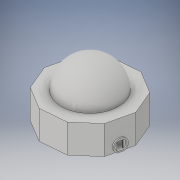
# Autodesk Inventor part: dome
Saved by Autodesk Inventor 2017 (Build 210142000, 142)
## iProperties
Created: 2018-03-05
Part Number: dome
Material: Generic
Document SubType Name: Modeling
Designer: Braxton
Density: 1 g/cm^3
Appearance: Default
Author: Braxton
Autodesk Inventor part; units mm, degrees
ref_plane "YZ Plane" through (0, 0, 0) normal (1, 0, 0) x (0, 1, 0)
ref_plane "XZ Plane" through (0, 0, 0) normal (0, 1, 0) x (-1, 0, 0)
ref_plane "XY Plane" through (0, 0, 0) normal (0, 0, 1) x (1, 0, 0)
sketch "Sketch1" plane through (0, 0, 0) normal (0, 1, 0) x (-1, 0, 0)
  line L0 (707.6587, -429.7359) -> (319.9155, -763.615)
  line L1 (319.9155, -763.615) -> (-190.0245, -805.8191)
  line L2 (-190.0245, -805.8191) -> (-627.3817, -540.2278)
  line L3 (-627.3817, -540.2278) -> (-825.1003, -68.2877)
  line L4 (-825.1003, -68.2877) -> (-707.6587, 429.7359)
  line L5 (-707.6587, 429.7359) -> (-319.9155, 763.615)
  line L6 (-319.9155, 763.615) -> (190.0245, 805.8191)
  line L7 (190.0245, 805.8191) -> (627.3817, 540.2278)
  line L8 (627.3817, 540.2278) -> (825.1003, 68.2877)
  line L9 (825.1003, 68.2877) -> (707.6587, -429.7359)
  point P0 (0, 0)
  point P1 (0, 0)
  dimension "d0" = 1574.8
  constraints: 20 end point, 1 coincident, 21 other
  measures "d0" distance between parallel lines of L5 L0
extrude "bace" add sketch "Sketch1" along normal blind 25.4
sketch "Sketch2" plane through (0, 25.4, 0) normal (0, 1, 0) x (1, 0, 0)
  line L0 (-319.9155, 763.615) -> (-707.6587, 429.7359) projected
  line L1 (-707.6587, 429.7359) -> (-319.9155, 763.615)
  line L2 (-319.9155, 763.615) -> (190.0245, 805.8191)
  line L3 (190.0245, 805.8191) -> (627.3817, 540.2278)
  line L4 (627.3817, 540.2278) -> (825.1003, 68.2877)
  line L5 (825.1003, 68.2877) -> (707.6587, -429.7359)
  line L6 (707.6587, -429.7359) -> (319.9155, -763.615)
  line L7 (319.9155, -763.615) -> (-190.0245, -805.8191)
  line L8 (-190.0245, -805.8191) -> (-627.3817, -540.2278)
  line L9 (-627.3817, -540.2278) -> (-825.1003, -68.2877)
  line L10 (-825.1003, -68.2877) -> (-707.6587, 429.7359)
  line L11 (-684.831, 415.8734) -> (-309.5957, 738.9822)
  line L12 (-309.5957, 738.9822) -> (183.8947, 779.825)
  line L13 (183.8947, 779.825) -> (607.1435, 522.8011)
  line L14 (607.1435, 522.8011) -> (798.4842, 66.0849)
  line L15 (798.4842, 66.0849) -> (684.831, -415.8734)
  line L16 (684.831, -415.8734) -> (309.5957, -738.9822)
  line L17 (309.5957, -738.9822) -> (-183.8947, -779.825)
  line L18 (-183.8947, -779.825) -> (-607.1435, -522.8011)
  line L19 (-607.1435, -522.8011) -> (-798.4842, -66.0849)
  line L20 (-798.4842, -66.0849) -> (-684.831, 415.8734)
  line L21 (-707.6587, 429.7359) -> (-825.1003, -68.2877) projected
  point P0 (0, 0)
  point P1 (0, 0)
  point P2 (0, 0)
  dimension "d4" = 25.4
  constraints: 40 end point, 2 coincident, 1 parallel, 42 other
  measures "d4" distance between parallel lines of L21 L20
extrude "bace wall" add sketch "Sketch2" along normal blind 508
sketch "Sketch3" plane through (0, 533.4, 0) normal (0, 1, 0) x (1, 0, 0)
  line L0 (-456.554, 277.2489) -> (-206.3971, 492.6548)
  line L1 (-206.3971, 492.6548) -> (122.5965, 519.8833)
  line L2 (122.5965, 519.8833) -> (404.7624, 348.534)
  line L3 (404.7624, 348.534) -> (532.3228, 44.0566)
  line L4 (532.3228, 44.0566) -> (456.554, -277.2489)
  line L5 (456.554, -277.2489) -> (206.3971, -492.6548)
  line L6 (206.3971, -492.6548) -> (-122.5965, -519.8833)
  line L7 (-122.5965, -519.8833) -> (-404.7624, -348.534)
  line L8 (-404.7624, -348.534) -> (-532.3228, -44.0566)
  line L9 (-532.3228, -44.0566) -> (-456.554, 277.2489)
  line L10 (-627.3817, -540.2278) -> (-825.1003, -68.2877) projected
  line L11 (-825.1003, -68.2877) -> (-707.6587, 429.7359)
  line L12 (-707.6587, 429.7359) -> (-319.9155, 763.615)
  line L13 (-319.9155, 763.615) -> (190.0245, 805.8191)
  line L14 (190.0245, 805.8191) -> (627.3817, 540.2278)
  line L15 (627.3817, 540.2278) -> (825.1003, 68.2877)
  line L16 (825.1003, 68.2877) -> (707.6587, -429.7359)
  line L17 (707.6587, -429.7359) -> (319.9155, -763.615)
  line L18 (319.9155, -763.615) -> (-190.0245, -805.8191)
  line L19 (-190.0245, -805.8191) -> (-627.3817, -540.2278)
  line L20 (-627.3817, -540.2278) -> (-825.1003, -68.2877)
  point P0 (0, 0)
  point P1 (0, 0)
  point P2 (-798.4842, -66.0849)
  point P3 (0, 0)
  point P4 (0, 0)
  dimension "d7" = 1016
  constraints: 40 end point, 2 coincident, 42 other
  measures "d7" distance between parallel lines of L4 L9
extrude "bace cieiling" add sketch "Sketch3" along normal blind 25.4
ref_plane "Work Plane1" through (-532.3228, 533.4, 44.0566) normal (-0.082481, 0, -0.9965926) x (0, 1, 0)
sketch "Sketch6" plane through (-532.3228, 533.4, 44.0566) normal (-0.082481, 0, -0.9965926) x (0, 1, 0)
  line L0 (25.4, 789.9846) -> (25.4, 278.301) projected
  line L1 (25.4, 0) -> (25.4, 102.0122) projected
  arc A0 (25.4, 0) -> (559.5428, 534.1428) centre (25.4, 534.1428) ccw
  line L2 (25.4, 534.1428) -> (559.5428, 534.1428) construction
  line L3 (25.4, 534.1428) -> (25.4, 0)
  arc A1 (25.4, -25.4) -> (584.9428, 534.1428) centre (25.4, 534.1428) ccw
  line L4 (25.4, 0) -> (25.4, -25.4)
  line L5 (559.5428, 534.1428) -> (584.9428, 534.1428)
  point P0 (-533.4, 534.1428)
  dimension "d12" = 25.4
  constraints: 8 end point, 4 point on circle, 2 centre point, 2 perpendicular, 1 coincident, 1 horizontal, 1 midpoint, 1 vertical
  measures "d12" radial gap between concentric circles of A0 A1
revolve "dome" add sketch "Sketch6" angle 360 about axis through (0, 558.8, 0) along (0, 1, 0)
sketch "Sketch8" plane through (825.1003, 0, -68.2877) normal (0.9733039, 0, 0.22952) x (0.22952, 0, -0.9733039)
  line L0 (-255.8418, 25.4) -> (-205.0418, 25.4)
  line L1 (-205.0418, 25.4) -> (-205.0418, 194.7333)
  line L2 (-205.0418, 194.7333) -> (-255.8418, 194.7333)
  line L3 (-255.8418, 194.7333) -> (-255.8418, 25.4)
  line L4 (-255.8418, 25.4) -> (-306.6418, 25.4)
  line L5 (-306.6418, 25.4) -> (-306.6418, 194.7333)
  line L6 (-306.6418, 194.7333) -> (-255.8418, 194.7333)
  line L7 (-503.4306, 25.4) -> (-8.253, 25.4) projected
  point P0 (-255.8418, 0)
  point P1 (-255.8418, 25.4)
  dimension "d16" = 50.8
  dimension "d17" = 169.3333
  constraints: 14 end point, 2 symmetric about line, 1 horizontal, 1 midpoint, 1 perpendicular
  measures "d16" distance of L0.start L0.end
  measures "d17" distance of L0.end L1.end
extrude "door frame" cut sketch "Sketch8" against normal blind 25.4
sketch "Sketch7" plane through (825.1003, 0, -68.2877) normal (0.9733039, 0, 0.22952) x (0.22952, 0, -0.9733039)
  line L0 (-306.6418, 194.7333) -> (-205.0418, 194.7333)
  line L1 (-306.6418, 25.4) -> (-205.0418, 25.4)
  arc A0 (-198.4359, 0) -> (-313.6926, 0.2332) centre (-255.8418, 110.0667) ccw
  arc A1 (-306.6418, 194.7333) -> (-306.6418, 25.4) centre (-255.8418, 110.0667) ccw
  arc A2 (-205.0418, 25.4) -> (-205.0418, 194.7333) centre (-255.8418, 110.0667) ccw
  line L2 (-306.6418, 194.7333) -> (-205.0418, 194.7333)
  line L3 (-306.6418, 194.7333) -> (-306.6418, 25.4)
  line L4 (-313.6926, 0.2332) -> (-198.4359, 0)
  point P0 (-255.8418, 0)
  point P1 (-255.8418, 194.7333)
  point P2 (-306.6418, 110.0667)
  point P3 (-255.8418, 110.0667)
  point P4 (-256.0642, 0.1166)
  dimension "d14" = 169.3333
  dimension "d15" = 101.6
  constraints: 10 end point, 6 point on circle, 3 centre point, 3 midpoint, 2 coincident, 1 horizontal, 1 parallel
  measures "d14" distance between parallel lines of L1 L0
  measures "d15" distance of L0.start L0.end
extrude "corridor connection" add sketch "Sketch7" along normal blind 25.4
sketch "Sketch9" plane through (729.998, 25.4, 224.3381) normal (0.22952, 0, -0.9733039) x (-0.9733039, 0, -0.22952)
  line L0 (-12.7, 169.3333) -> (-6.35, 169.3333)
  line L1 (-6.35, 169.3333) -> (-6.35, 0)
  line L2 (-6.35, 0) -> (-19.05, 0)
  line L3 (-19.05, 0) -> (-19.05, 169.3333)
  line L4 (-12.7, 169.3333) -> (-19.05, 169.3333)
  line L5 (-25.4, -25.4) -> (-25.4, 208.8041) projected
  point P0 (762, -25.4)
  point P1 (-25.4, -25.4)
  point P2 (-25.4, 169.3333)
  point P3 (0, 169.3333)
  point P4 (-25.4, 0)
  point P5 (0, 0)
  point P6 (-25.4, 169.3333)
  point P7 (-25.4, -25.1668)
  dimension "d22" = 6.35
  dimension "d23" = 12.7
  dimension "d24" = 169.3333
  constraints: 10 end point, 1 point on line
  measures "d22" distance of L0.start L0.end
  measures "d23" distance of L1.end L2.end
  measures "d24" distance between parallel lines of L2 L0
extrude "left door slot" cut sketch "Sketch9" against normal blind 50.8
ref_plane "door slot mirror" through (766.3795, 25.4, 180.7241) normal (0.22952, 0, -0.9733039) x (-0.9733039, 0, -0.22952)
mirror "Mirror1" about plane through (766.3795, 25.4, 180.7241) normal (0.22952, 0, -0.9733039) of "left door slot"
ref_plane "terminal connection workplane" through (-2480.0562, 0, -584.8353) normal (-0.22952, 0, 0.9733039) x (0, 1, 0)
body "Solid1"
